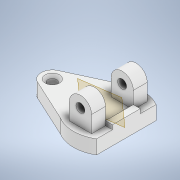
# Autodesk Inventor part: Part10
Saved by Autodesk Inventor 2022.3 (Build 263350000, 350)
## iProperties
Created: 2022-11-16
Part Number: Part10
Material: PC/ABS Plastic
Document SubType Name: Modeling
Designer: komputer
Density: 0.357273 g/cm^3
Appearance: Smooth - White
Mass: 1.17867 g
Surface Area: 21.625 cm^2
Volume: 3.29908 cm^3
Author: komputer
Autodesk Inventor part; units mm, degrees
ref_plane "YZ Plane" through (0, 0, 0) normal (1, 0, 0) x (0, 1, 0)
ref_plane "XZ Plane" through (0, 0, 0) normal (0, 1, 0) x (-1, 0, 0)
ref_plane "XY Plane" through (0, 0, 0) normal (0, 0, 1) x (1, 0, 0)
sketch "Sketch1" plane through (0, 0, 0) normal (0, 1, 0) x (-1, 0, 0)
  circle A0 centre (0, 0) radius 12.5
  dimension "d0" = 25
  constraints: 1 centre point, 1 coincident
  measures "d0" diameter of A0
extrude "Extrusion1" add sketch "Sketch1" along normal blind 5
sketch "Sketch2" plane through (0, 5, 0) normal (0, 1, 0) x (1, 0, 0)
  line L0 (0, 5) -> (0, -5)
  line L1 (0, -5) -> (-4, -5)
  line L2 (-4, -5) -> (-4, 5)
  line L3 (-4, 5) -> (0, 5)
  line L4 (0, 5) -> (0, -5)
  line L5 (0, -5) -> (4, -5)
  line L6 (4, -5) -> (4, 5)
  line L7 (4, 5) -> (0, 5)
  line L8 (0, 5) -> (0, -5)
  line L9 (4, -5) -> (-4, -5)
  line L10 (-4, -5) -> (-4, -10)
  line L11 (-4, -10) -> (4, -10)
  line L12 (4, -10) -> (4, -5)
  line L13 (4, 5) -> (-4, 5)
  line L14 (-4, 5) -> (-4, 10)
  line L15 (-4, 10) -> (4, 10)
  line L16 (4, 10) -> (4, 5)
  point P0 (0, 0)
  dimension "d4" = 10
  dimension "d5" = 4
  dimension "d6" = 4
  dimension "d7" = 5
  dimension "d8" = 5
  constraints: 34 end point, 8 parallel, 4 horizontal, 4 perpendicular, 1 point on line
  measures "d4" distance of L0.start L0.end
  measures "d5" distance of L2.end L3.end
  measures "d6" distance of L7.end L6.end
  measures "d7" distance of L10.end L9.end
  measures "d8" distance of L13.end L14.end
extrude "Extrusion2" add sketch "Sketch2" along normal blind 10 contours L3 L14 L15 L16 L7 | L5 L12 L11 L10 L1
sketch "Sketch3" plane through (-4, 5, 10) normal (0, 0, 1) x (1, 0, 0)
  line L0 (0, 10) -> (8, 10) projected
  line L1 (0, 0) -> (0, 10) projected
  line L2 (8, 0) -> (8, 10) projected
  circle A0 centre (4, 6) radius 4
  circle A1 centre (4, 6) radius 1.6
  point P0 (4, -5)
  point P1 (0, 6)
  point P2 (4, 10)
  point P3 (8, 6)
  dimension "d11" = 3.2
  constraints: 3 tangent, 2 centre point, 1 coincident
  measures "d11" diameter of A1
extrude "Extrusion3" cut sketch "Sketch3" against normal through all contours L0 A0 L1 | L0 L2 A0 | A1
sketch "Sketch4" plane through (0, 5, 0) normal (0, 1, 0) x (1, 0, 0)
  circle A0 centre (0, 0) radius 12.5 projected
  line L0 (4, -5) -> (4, -10) projected
  line L1 (4, -10) -> (14.8106, -10)
  line L2 (14.8106, -10) -> (14.8106, 15.6874)
  line L3 (14.8106, 15.6874) -> (4, 15.6874)
  line L4 (4, 15.6874) -> (4, -10)
  line L5 (14.8106, 15.6874) -> (4, 15.6874)
  line L6 (4, 15.6874) -> (4, -20.4825)
  line L7 (4, -20.4825) -> (14.8106, -20.4825)
  line L8 (14.8106, -20.4825) -> (14.8106, 15.6874)
  line L9 (4, 15.6874) -> (6.5, 15.6874)
  line L10 (6.5, 15.6874) -> (6.5, -20.4825)
  line L11 (6.5, -20.4825) -> (4, -20.4825)
  line L12 (4, -20.4825) -> (4, 15.6874)
  point P0 (6.5, 10.6771)
  point P1 (6.5, -10.6771)
  dimension "d14" = 2.5
  constraints: 24 end point, 6 parallel, 3 horizontal, 3 perpendicular, 2 point on line
  measures "d14" distance of L10.end L11.end
extrude "Extrusion4" cut sketch "Sketch4" against normal blind 10 contours A0 L1 L10 | A0 L10 L1
sketch "Sketch5" plane through (0, 0, 0) normal (0, -1, 0) x (1, 0, 0)
  line L0 (6.5, -10.6771) -> (6.5, 10.6771) projected
  arc A0 (6.5, 10.6771) -> (6.5, -10.6771) centre (0, 0) ccw projected
  line L1 (0, 0) -> (-29.6517, 0)
  line L2 (-29.6517, 0) -> (-6.5, 10.6771)
  arc A1 (6.5, 10.6771) -> (6.5, -10.6771) centre (0, 0) ccw projected
  line L3 (-29.6517, 0) -> (-6.5, -10.6771)
  point P0 (-6.5, 10.6771)
  constraints: 6 end point, 2 point on circle, 1 horizontal
extrude "Extrusion5" add sketch "Sketch5" against normal blind 5 contours L3 L1 A0 | A0 L1 L2
fillet "Fillet1" radius 4 1 edges at (-29.6517, 2.5, 0)
sketch "Sketch6" plane through (0, 5, 0) normal (0, 1, 0) x (1, 0, 0)
  arc A0 (-21.7755, 3.6323) -> (-21.7755, -3.6323) centre (-20.1004, 0) ccw projected
  line L0 (-21.7755, -3.6323) -> (-6.5, -10.6771) projected
  arc A1 (-6.5, -10.6771) -> (6.5, -10.6771) centre (0, 0) ccw projected
  line L1 (6.5, -10.6771) -> (6.5, 10.6771) projected
  arc A2 (6.5, 10.6771) -> (-6.5, 10.6771) centre (0, 0) ccw projected
  line L2 (-6.5, 10.6771) -> (-21.7755, 3.6323) projected
  line L3 (4, -5) -> (4, -10) projected
  line L4 (4, -10) -> (-4, -10) projected
  line L5 (-4, -10) -> (-4, -5) projected
  line L6 (-4, -5) -> (4, -5) projected
  line L7 (4, 10) -> (4, 5) projected
  line L8 (4, 5) -> (-4, 5) projected
  line L9 (-4, 5) -> (-4, 10) projected
  line L10 (-4, 10) -> (4, 10) projected
  circle A3 centre (-20.1004, 0) radius 1.6
  circle A4 centre (-5.1349, 0) radius 1.6
  dimension "d20" = 3.2
  dimension "d21" = 3.2
  constraints: 2 centre point, 1 coincident
  measures "d20" diameter of A3
  measures "d21" diameter of A4
extrude "Extrusion6" cut sketch "Sketch6" against normal blind 10 contours A3 | A4
chamfer "Chamfer1" distance 1 angle 45 2 edges at (-21.7004, 5, 0) (-6.7349, 5, 0)
ref_plane "Work Plane1" through (11.4116, 8.3973, 5) normal (0, 0, 1) x (-0.1242072, 0.9922563, 0)
sketch "Sketch8" plane through (11.4116, 8.3973, 5) normal (0, 0, 1) x (-0.1242072, 0.9922563, 0)
  line L0 (-1.1462, 18.1949) -> (-6.1075, 18.8159) projected
  line L1 (-6.1075, 18.8159) -> (-7.7222, 5.9166) projected
  line L2 (-7.7222, 5.9166) -> (-2.7609, 5.2956) projected
  line L3 (-1.1462, 18.1949) -> (-2.7609, 5.2956) projected
  arc A0 (3.5032, 7.031) -> (4.4968, 14.969) centre (4, 11) ccw projected
  line L4 (-1.4567, 15.7143) -> (4.4968, 14.969) projected
  line L5 (-2.4504, 7.7762) -> (-1.4567, 15.7143) projected
  line L6 (-2.4504, 7.7762) -> (3.5032, 7.031) projected
  circle A1 centre (4, 11) radius 1.6 projected
  line L7 (0, 2) -> (8, 2) projected
  line L8 (8, 2) -> (8, 11) projected
  arc A2 (8, 11) -> (0, 11) centre (4, 11) ccw projected
  line L9 (0, 2) -> (0, 11) projected
  circle A3 centre (4, 11) radius 1.65 projected
  line L10 (-2.7609, 5.2956) -> (0, 4.95)
  line L11 (0, 4.95) -> (0, 15.5319)
  point P0 (-6.9148, 12.3663)
  point P1 (0, 11)
  point P2 (-1.4567, 15.7143)
  constraints: 4 end point, 3 point on line
extrude "Extrusion7" add sketch "Sketch8" against normal up to surface (10 mm away) contours L4 L11 L9 L6 L3 | L6 L9 L10 L3
sketch "Sketch9" plane through (0, 11, -5) normal (0, 0, 1) x (1, 0, 0)
  circle A0 centre (0, 0) radius 1.6 projected
  line L0 (-4, -4.5319) -> (4, -3.5305) projected
  line L1 (4, -3.5305) -> (4, 0) projected
  arc A1 (4, 0) -> (-4, 0) centre (0, 0) ccw projected
  line L2 (-4, -4.5319) -> (-4, 0) projected
  arc A2 (4, 0) -> (-4, 0) centre (0, 0) ccw projected
  line L3 (-4, -6) -> (-4, 0) projected
  line L4 (4, -6) -> (-4, -6) projected
  line L5 (4, -6) -> (4, 0) projected
  circle A3 centre (0, 0) radius 1.6 projected
  point P0 (0, -11)
  point P1 (4, -3.5305)
extrude "Extrusion8" cut sketch "Sketch9" along normal up to surface (10 mm away) contours L0 L5 L4 L3
sketch "Sketch10" plane through (11.4116, 8.3973, 5) normal (0, 0, 1) x (0.9922563, 0.1242072, 0)
  line L0 (-7.7762, -2.4504) -> (-7.4695, 0) projected
  line L1 (-5.2956, -2.7609) -> (-7.7762, -2.4504) projected
  line L2 (-5.2956, -2.7609) -> (-4.95, 0) projected
  line L3 (-4.95, 0) -> (-7.4695, 0) projected
  line L4 (-5.2956, -2.7609) -> (-4.95, 0) projected
  line L5 (-5.1033, -1.2252) -> (-7.584, -0.9147)
  line L6 (-7.7762, -2.4504) -> (-7.031, 3.5032) projected
  point P0 (-12.3663, -6.9148)
  point P1 (-7.584, -0.9147)
  point P2 (-5.1033, -1.2252)
  constraints: 2 end point, 2 point on line, 1 perpendicular
extrude "Extrusion9" cut sketch "Sketch10" against normal blind 10 contours L0 L3 L2 L5
body "Solid1"
